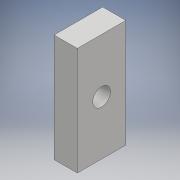
# Autodesk Inventor part: GPU Clamp
Saved by Autodesk Inventor 2017 (Build 210142000, 142)
## iProperties
Created: 2019-06-29
Part Number: GPU Clamp
Material: Generic
Document SubType Name: Modeling
Designer: DDeGo
Density: 1 g/cm^3
Appearance: Default
Author: DDeGo
Autodesk Inventor part; units mm, degrees
ref_plane "YZ Plane" through (0, 0, 0) normal (1, 0, 0) x (0, 1, 0)
ref_plane "XZ Plane" through (0, 0, 0) normal (0, 1, 0) x (-1, 0, 0)
ref_plane "XY Plane" through (0, 0, 0) normal (0, 0, 1) x (1, 0, 0)
sketch "Sketch1" plane through (0, 0, 0) normal (1, 0, 0) x (0, 1, 0)
  line L0 (-4.5, 10) -> (4.5, 10)
  line L1 (4.5, 10) -> (4.5, -10)
  line L2 (4.5, -10) -> (-4.5, -10)
  line L3 (-4.5, -10) -> (-4.5, 10)
  line L4 (-4.5, 10) -> (4.5, -10) construction
  line L5 (4.5, 10) -> (-4.5, -10) construction
  circle A0 centre (0, 0) radius 1.65
  point P0 (0, 0)
  dimension "d0" = 9
  dimension "d1" = 20
  dimension "d2" = 3.3
  constraints: 12 end point, 4 midpoint, 2 parallel, 1 centre point, 1 horizontal, 1 perpendicular
  measures "d0" distance of L1.end L2.end
  measures "d1" distance of L0.end L1.end
  measures "d2" diameter of A0
extrude "Extrusion1" add sketch "Sketch1" along normal blind 4.3
body "Solid1"
